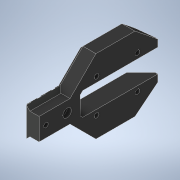
# Autodesk Inventor part: Underrail
Saved by Autodesk Inventor 2021 (Build 250183000, 183)
## iProperties
Created: 2024-08-02
Part Number: Underrail
Material: Generic
Document SubType Name: Modeling
Designer: Lukas
Density: 1 g/cm^3
Appearance: Default
Author: Lukas
Autodesk Inventor part; units mm, degrees
ref_plane "YZ Plane" through (0, 0, 0) normal (1, 0, 0) x (0, 1, 0)
ref_plane "XZ Plane" through (0, 0, 0) normal (0, 1, 0) x (-1, 0, 0)
ref_plane "XY Plane" through (0, 0, 0) normal (0, 0, 1) x (1, 0, 0)
sketch "Sketch1" plane through (0, 0, 0) normal (1, 0, 0) x (0, 1, 0)
  circle A0 centre (12, 16.725) radius 1.6
  circle A1 centre (-12, 16.725) radius 1.6
  circle A2 centre (-12, -12.275) radius 1.6
  circle A3 centre (12, -12.275) radius 1.6
  line L0 (-8.25, -26.675) -> (-8.25, 26.675)
  line L1 (-8.25, 26.675) -> (-6.4, 28.525)
  line L2 (-6.4, 28.525) -> (6.4, 28.525)
  line L3 (6.4, 28.525) -> (8.25, 26.675)
  line L4 (8.25, 26.675) -> (8.25, -26.675)
  line L5 (-26.25, -10.4251) -> (-26.25, 51.5125)
  line L6 (-26.25, 51.5125) -> (-16, 57.725)
  line L7 (-16, 57.725) -> (16, 57.725)
  line L8 (16, 57.725) -> (26.25, 51.5125)
  line L9 (26.25, 51.5125) -> (26.25, -10.4251)
  line L10 (-8.25, -26.675) -> (-13.25, -26.675)
  line L11 (-13.25, -26.675) -> (-26.25, -10.4251)
  line L12 (8.25, -26.675) -> (13.25, -26.675)
  line L13 (13.25, -26.675) -> (26.25, -10.4251)
  point P0 (0, 0)
  point P1 (0, -20.7974)
  point P2 (0, 28.525)
  point P3 (-8.25, 0)
  point P4 (0, 57.725)
  dimension "d0" = 24
  dimension "d1" = 29
  dimension "d2" = 16.5
  dimension "d3" = 12
  dimension "d4" = 3.2
  dimension "d5" = 11.8
  dimension "d6" = 1.85
  dimension "d7" = 1.85
  dimension "d9" = 55.2
  dimension "d11" = 29.2
  dimension "d12" = 148.78
  dimension "d13" = 32
  dimension "d16" = 18
  dimension "d17" = 5
  dimension "d19" = 141.34
  constraints: 28 end point, 5 horizontal alignment, 5 vertical alignment, 4 centre point, 4 equal length, 3 equal radius, 3 midpoint, 2 parallel, 2 perpendicular, 2 vertical, 1 horizontal, 1 point on line
  measures "d0" distance of A0.centre A1.centre
  measures "d1" distance of A2.centre A1.centre
  measures "d2" distance between parallel lines of L4 L0
  measures "d3" horizontal distance of point (0, 0) A2.centre
  measures "d4" diameter of A2
  measures "d5" distance from line of A1.centre L2
  measures "d6" horizontal distance of L0.end L1.end
  measures "d7" horizontal distance of L0.end L1.end
  measures "d9" distance from line of L2 L4.end
  measures "d11" distance between parallel lines of L7 L2
  measures "d12" angle of L8 L7
  measures "d13" distance of L6.end L7.end
  measures "d16" distance between parallel lines of L5 L0
  measures "d17" distance of L0.start L10.end
  measures "d19" angle of L11 L5
extrude "Extrusion1" add sketch "Sketch1" along normal blind 12
sketch "Sketch2" plane through (0, -16, 57.725) normal (0, 0, 1) x (1, 0, 0)
  line L0 (0, 42.25) -> (12, 42.25) projected
  line L1 (0, -10.25) -> (12, -10.25) projected
  line L2 (9.32, 56) -> (9.32, 23.8368)
  line L3 (9.32, 23.8368) -> (5.54, 23.8368)
  line L4 (5.54, 23.8368) -> (2.77, 26.6059)
  line L5 (2.77, 26.6059) -> (0, 23.835)
  line L6 (0, 8.165) -> (2.77, 5.3959)
  line L7 (2.77, 5.3959) -> (5.54, 8.165)
  line L8 (5.54, 8.165) -> (9.32, 8.165)
  line L9 (9.32, 8.165) -> (9.32, -24)
  line L10 (9.32, -24) -> (-10.68, -24)
  line L11 (-10.68, -24) -> (-10.68, 56)
  line L12 (-10.68, 56) -> (9.32, 56)
  line L13 (0, 32) -> (0, 0) projected
  line L14 (0, 23.835) -> (0, 21.075)
  line L15 (0, 22.4) -> (12, 22.4) projected
  line L16 (0, 21.075) -> (0, 21.075)
  line L17 (0, 21.075) -> (0, 10.925)
  line L18 (0, 10.925) -> (0, 10.925)
  line L19 (0, 10.925) -> (0, 8.165)
  point P0 (0, 16)
  point P1 (5, 42.25)
  point P2 (5, -10.25)
  point P3 (0, 16)
  point P4 (-10.68, 16)
  point P5 (0, 16)
  point P6 (0, 16)
  point P7 (0, 16)
  dimension "d23" = 15.6718
  dimension "d29" = 15.67
  dimension "d30" = 2.76
  dimension "d32" = 10.15
  dimension "d33" = 2.77
  dimension "d34" = 2.77
  dimension "d35" = 3.78
  dimension "d36" = 0
  dimension "d37" = 20
  dimension "d38" = 80
  constraints: 32 end point, 10 perpendicular, 5 midpoint, 4 point on line, 2 equal length, 2 vertical, 2 vertical alignment, 1 coincident, 1 horizontal alignment, 1 parallel
  measures "d23" distance between parallel lines of L8 L3
  measures "d29" distance of L6.start L5.end
  measures "d30" distance of L5.end L14.end
  measures "d32" distance of L16.end L17.end
  measures "d33" horizontal distance of L4.end L5.end
  measures "d34" horizontal distance of L3.end L4.end
  measures "d35" distance of L2.end L3.end
  measures "d36" distance of L14.end L16.end
  measures "d37" distance of L9.end L10.end
  measures "d38" distance of L10.end L11.end
extrude "Extrusion2" cut sketch "Sketch2" against normal blind 22
chamfer "Chamfer3" distance 18.415 angle 45 2 edges at (4.66, 26.25, 35.725) (4.66, -26.25, 35.725)
chamfer "Chamfer2" distance 2.77 angle 45 6 edges at (0, 17.0425, 26.5175) (0, -17.0425, 26.5175) (0, -26.25, 3.4425) (0, 26.25, 3.4425) (0, -19.75, -18.5501) (0, 19.75, -18.5501)
sketch "Sketch3" plane through (9.32, 7.8368, 57.725) normal (-1, 0, 0) x (0, 0, 1)
  line L0 (-6.2125, 18.4132) -> (0, 8.1632) projected
  line L1 (-40.415, 18.4132) -> (-6.2125, 18.4132) projected
  line L2 (0, 0) -> (-22.0018, 0) projected
  line L3 (0, 8.1632) -> (0, 0) projected
  line L4 (0, -23.8368) -> (-6.2125, -34.0868) projected
  line L5 (0, -15.6718) -> (0, -23.8368) projected
  line L6 (0, -15.6718) -> (-22, -15.6718) projected
  line L7 (-22, -15.6718) -> (-22, -15.6718) projected
  line L8 (-6.2125, -34.0868) -> (-40.415, -34.0868) projected
  line L9 (-40.415, -34.0868) -> (-22, -15.6718) projected
  line L10 (-40.415, 18.4132) -> (-22.0018, 0) projected
  point P0 (-57.725, -7.8368)
extrude "Extrusion3" cut sketch "Sketch3" against normal through all
sketch "Sketch4" plane through (0, 0, 0) normal (0, 1, 0) x (-1, 0, 0)
  line L0 (1, 39.725) -> (-3, 39.725)
  line L1 (-3, 39.725) -> (-3, 34.475)
  line L2 (-3, 34.475) -> (1, 34.475)
  line L3 (1, 34.475) -> (1, 39.725)
  line L4 (0, 31.8076) -> (0, 57.725) projected
  line L5 (-5.54, 57.725) -> (-12, 57.725) projected
  point P0 (0, 0)
  dimension "d56" = 5.25
  dimension "d58" = 4
  dimension "d64" = 1
  dimension "d65" = 18
  constraints: 8 end point, 2 parallel, 1 horizontal, 1 perpendicular
  measures "d56" distance of L2.end L0.start
  measures "d58" distance of L1.end L2.end
  measures "d64" distance between parallel lines of L4 L3
  measures "d65" distance between parallel lines of L5 L0
extrude "Extrusion4" cut sketch "Sketch4" along normal through all both and the other way through all
pattern_linear "Rectangular Pattern1" count 3 spacing 10 along (0, 0, 1) of "Extrusion4"
sketch "Sketch5" plane through (12, 0, 0) normal (1, 0, 0) x (0, 0, -1)
  circle A0 centre (-37.725, 0.0009) radius 3
  circle A1 centre (-52.725, 0.0009) radius 1.6
  line L0 (-57.725, 7.8368) -> (-57.725, -7.835) projected
  point P0 (0, 0)
  point P1 (-57.725, 0.0009)
  dimension "d66" = 5
  dimension "d67" = 20
  dimension "d68" = 6
  dimension "d69" = 3.2
  constraints: 2 centre point, 2 horizontal alignment, 1 midpoint
  measures "d66" distance from line of L0 A1.centre
  measures "d67" distance from line of L0 A0.centre
  measures "d68" diameter of A0
  measures "d69" diameter of A1
extrude "Extrusion5" cut sketch "Sketch5" against normal blind 3 contours A0
extrude "Extrusion6" cut sketch "Sketch5" against normal through all contours A1
sketch "Sketch6" plane through (0, 0, 0) normal (-1, 0, 0) x (0, 0, 1)
  circle A0 centre (52.725, 0.0009) radius 1.6 projected
  circle A1 centre (52.725, 0.0009) radius 1.6 projected
  circle A2 centre (52.725, 0.0009) radius 3
  circle A3 centre (16.725, -12) radius 1.6 projected
  circle A4 centre (-12.275, -12) radius 1.6 projected
  circle A5 centre (-12.275, 12) radius 1.6 projected
  circle A6 centre (16.725, 12) radius 1.6 projected
  circle A7 centre (16.725, -12) radius 3
  circle A8 centre (-12.275, -12) radius 3
  circle A9 centre (-12.275, 12) radius 3
  circle A10 centre (16.725, 12) radius 3
  point P0 (0, 0)
  dimension "d74" = 6
  constraints: 5 centre point, 5 coincident, 4 equal radius
  measures "d74" diameter of A2
extrude "Extrusion7" cut sketch "Sketch6" against normal blind 9
chamfer "Chamfer5" distance 10 angle 45 2 edges at (0, -8.9763, -26.675) (0, 8.9763, -26.675)
equation "\"d3\" = 0.5 * d0"
equation "\"d7\" = d6"
body "Solid1"
